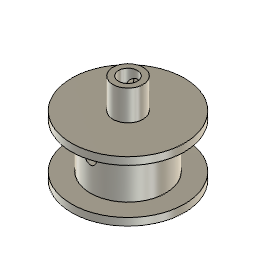
spool (Autodesk Fusion 360 design; units mm, degrees)
Autodesk Fusion 360 part; units mm, degrees
sketch "Sketch1" plane through (0, 0, 0) normal (0, 0, 1) x (1, 0, 0)
  circle A0 centre (0, 0) radius 15
  dimension "d1" = 30
  constraint coincident A0.centre origin
  measures "d1" diameter of A0
extrude "Extrude1" add sketch "Sketch1" along normal blind 16
ref_plane "WorkPlane2" through (0, 0, 2) normal (0, 0, 1) x (1, 0, 0)
sketch "Sketch2" plane through (0, 0, 2) normal (0, 0, 1) x (1, 0, 0)
  circle A0 centre (0, 0) radius 10
  circle A1 centre (0, 0) radius 15
  dimension "d6" = 20
  constraint coincident A0.centre A1.centre
  measures "d6" diameter of A0
extrude "Extrude2" cut sketch "Sketch2" along normal blind 12
sketch "Sketch3" plane through (0, 0, 16) normal (0, 0, 1) x (-1, 0, 0)
  circle A0 centre (0, 0) radius 15
  circle A1 centre (0, 0) radius 4
  dimension "d9" = 8
  constraint coincident A0.centre A1.centre
  measures "d9" diameter of A1
extrude "Extrude3" add sketch "Sketch3" along normal blind 8 contours A1
sketch "Sketch4" plane through (0, 0, 0) normal (0, 1, 0) x (1, 0, 0)
  circle A0 centre (0, -20) radius 2
  circle A1 centre (0, -10) radius 1.5
  dimension "d12" = 4
  dimension "d13" = 3
  measures "d12" diameter of A0
  measures "d13" diameter of A1
extrude "Extrude4" cut sketch "Sketch4" along normal blind 5 contours A0
extrude "Extrude5" cut sketch "Sketch4" along normal mid plane 40 contours A1
sketch "Sketch5" plane through (0, 0, 24) normal (0, 0, 1) x (-1, 0, 0)
  circle A0 centre (0, 0) radius 4
  circle A1 centre (0, 0) radius 2.5
  dimension "d18" = 5
  constraint concentric A0 A1
  measures "d18" diameter of A1
extrude "Extrude6" cut sketch "Sketch5" against normal blind 10 contours A1
